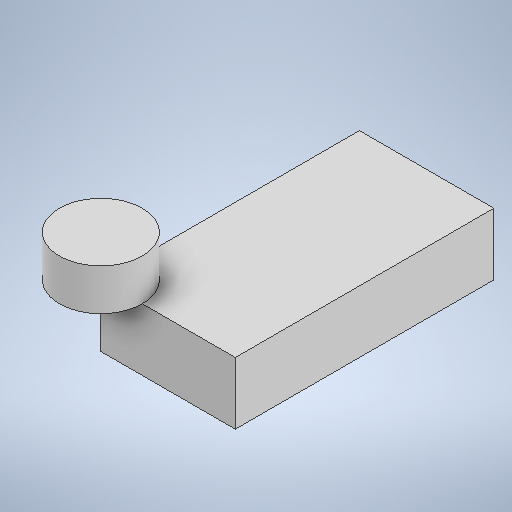
# Autodesk Inventor part: Sensor_VL53L1X
Saved by Autodesk Inventor 2025 (Build 290162000, 162)
## iProperties
Created: 2026-06-16
Part Number: Sensor_VL53L1X
Material: Generisch
Document SubType Name: Modeling
Designer: GemmiDad-GBSE
Density: 1 g/cm^3
Appearance: Vorgabe
Author: GemmiDad-GBSE
Autodesk Inventor part; units mm, degrees
ref_plane "YZ Plane" through (0, 0, 0) normal (1, 0, 0) x (0, 1, 0)
ref_plane "XZ Plane" through (0, 0, 0) normal (0, 1, 0) x (-1, 0, 0)
sketch "Skizze1" plane through (0, 0, 0) normal (0, 0, 1) x (1, 0, 0)
  line L0 (0, 0) -> (6.5, 0)
  line L1 (6.5, 0) -> (6.5, 12.5)
  line L2 (6.5, 12.5) -> (0, 12.5)
  line L3 (0, 12.5) -> (0, 0)
  constraints: 8 end point, 2 parallel, 1 horizontal, 1 perpendicular
extrude "Extrusion1" add sketch "Skizze1" along normal blind 3
ref_plane "Arbeitsebene1" through (0, 0, 3) normal (0, 0, 1) x (1, 0, 0)
sketch "Skizze2" plane through (0, 0, 3) normal (0, 0, 1) x (1, 0, 0)
  circle A0 centre (0, 0) radius 2
  constraints: 1 centre point
extrude "Extrusion2" add sketch "Skizze2" along normal blind 2 separate body
